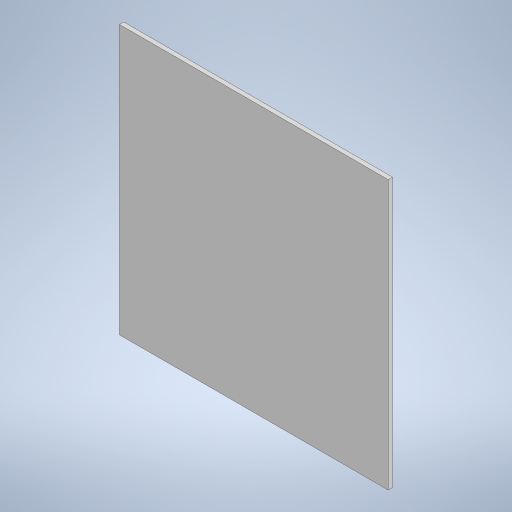
# Autodesk Inventor part: Part7
Saved by Autodesk Inventor 2023 (Build 270158000, 158)
## iProperties
Created: 2024-03-19
Part Number: Part7
Material: Generic
Document SubType Name: Modeling
Designer: noname
Density: 1 g/cm^3
Appearance: Default
Author: noname
Autodesk Inventor part; units mm, degrees
ref_plane "YZ Plane" through (0, 0, 0) normal (1, 0, 0) x (0, 1, 0)
ref_plane "XZ Plane" through (0, 0, 0) normal (0, 1, 0) x (-1, 0, 0)
ref_plane "XY Plane" through (0, 0, 0) normal (0, 0, 1) x (1, 0, 0)
sketch "Sketch1" plane through (0, 0, 0) normal (0, 0, 1) x (1, 0, 0)
  line L0 (-58.5, 42.5) -> (-58.5, -47.5) projected
  line L1 (-58.5, -47.5) -> (41.5, -47.5) projected
  line L2 (41.5, -47.5) -> (41.5, 42.5) projected
  line L3 (41.5, 42.5) -> (-58.5, 42.5) projected
  line L4 (-58.5, 42.5) -> (41.5, 42.5)
  line L5 (41.5, 42.5) -> (41.5, -57.5)
  line L6 (41.5, -57.5) -> (-58.5, -57.5)
  line L7 (-58.5, -57.5) -> (-58.5, 42.5)
  line L8 (42.73, 26.5) -> (60.73, 26.5)
  line L9 (60.73, 26.5) -> (60.73, 8.5)
  line L10 (60.73, 8.5) -> (42.73, 8.5)
  line L11 (42.73, 8.5) -> (42.73, 26.5)
  line L12 (42.73, -11.5) -> (42.73, 6.5)
  line L13 (60.73, -11.5) -> (42.73, -11.5)
  line L14 (60.73, 6.5) -> (60.73, -11.5)
  line L15 (42.73, 6.5) -> (60.73, 6.5)
  line L16 (42.73, -31.5) -> (42.73, -13.5)
  line L17 (60.73, -31.5) -> (42.73, -31.5)
  line L18 (60.73, -13.5) -> (60.73, -31.5)
  line L19 (42.73, -13.5) -> (60.73, -13.5)
  line L20 (41.5, 42.5) -> (41.5, 27.4671)
  line L21 (41.5, 27.4671) -> (41.5, -32.4671)
  line L22 (41.5, -32.4671) -> (41.5, -47.5)
  line L23 (-4, -34.5) -> (-13, -34.5) projected
  line L24 (-13, -34.5) -> (-13, 32.5) projected
  line L25 (-13, 32.5) -> (-4, 32.5) projected
  line L26 (-4, 32.5) -> (-4, -34.5) projected
  line L27 (-23, -34.5) -> (-32, -34.5) projected
  line L28 (-32, -34.5) -> (-32, 32.5) projected
  line L29 (-32, 32.5) -> (-23, 32.5) projected
  line L30 (-23, 32.5) -> (-23, -34.5) projected
  line L31 (15, -34.5) -> (6, -34.5) projected
  line L32 (6, -34.5) -> (6, 32.5) projected
  line L33 (6, 32.5) -> (15, 32.5) projected
  line L34 (15, 32.5) -> (15, -34.5) projected
  line L35 (-42, -34.5) -> (-51, -34.5) projected
  line L36 (-51, -34.5) -> (-51, 32.5) projected
  line L37 (-51, 32.5) -> (-42, 32.5) projected
  line L38 (-42, 32.5) -> (-42, -34.5) projected
  line L39 (34, -34.5) -> (25, -34.5) projected
  line L40 (25, -34.5) -> (25, 32.5) projected
  line L41 (25, 32.5) -> (34, 32.5) projected
  line L42 (34, 32.5) -> (34, -34.5) projected
  point P0 (0, 0)
  point P1 (-38.5, -35)
  point P2 (-41.5, -35)
  point P3 (-41.5, 32)
  point P4 (-38.5, 32)
  point P5 (-20.5, -35)
  point P6 (-23.5, -35)
  point P7 (-23.5, 32)
  point P8 (-20.5, 32)
  point P9 (-2.5, -35)
  point P10 (-5.5, -35)
  point P11 (-5.5, 32)
  point P12 (-2.5, 32)
  point P13 (15.5, -35)
  point P14 (12.5, -35)
  point P15 (12.5, 32)
  point P16 (15.5, 32)
  point P17 (33.5, -35)
  point P18 (30.5, -35)
  point P19 (30.5, 32)
  point P20 (33.5, 32)
  point P21 (41.5, -47.5)
  point P22 (-58.5, -47.5)
  point P23 (41.5, -2.5)
  dimension "d0" = 100
  dimension "d6" = 20
  constraints: 38 end point, 4 parallel, 2 equal length, 2 horizontal, 2 perpendicular, 2 vertical, 1 midpoint, 26 other
  measures "d0" distance between parallel lines of L6 L3
  measures "d6" distance of L8.start L12.end
extrude "Extrusion1" add sketch "Sketch1" along normal blind 1.6 contours L3 L2 L1 L0 | L1 L5 L6 L7 | L23 L24 L25 L26 | L27 L28 L29 L30 | L31 L32 L33 L34 | L35 L36 L37 L38 | L39 L40 L41 L42
body "Solid1"
